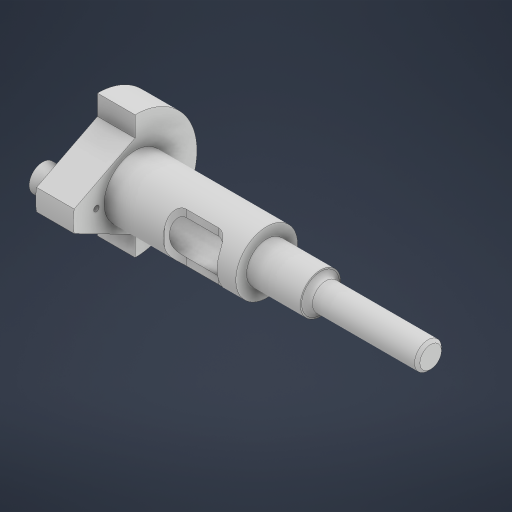
# Autodesk Inventor part: Part4
Saved by Autodesk Inventor 2023 (Build 270158000, 158)
## iProperties
Created: 2023-04-25
Part Number: Part4
Material: Ogólny
Document SubType Name: Modeling
Designer: Adam
Density: 1 g/cm^3
Appearance: Domyślna
Author: Adam
Autodesk Inventor part; units mm, degrees
ref_plane "YZ Plane" through (0, 0, 0) normal (1, 0, 0) x (0, 1, 0)
ref_plane "XZ Plane" through (0, 0, 0) normal (0, 1, 0) x (-1, 0, 0)
ref_plane "XY Plane" through (0, 0, 0) normal (0, 0, 1) x (1, 0, 0)
sketch "Szkic1" plane through (0, 0, 0) normal (0, 0, 1) x (1, 0, 0)
  line L0 (0, 0) -> (14, 0)
  line L1 (14, 0) -> (14, 23)
  line L2 (14, 23) -> (0, 23)
  line L3 (0, 23) -> (0, 0)
  line L4 (14, 0) -> (63, 0)
  line L5 (63, 0) -> (63, 11.5)
  line L6 (63, 11.5) -> (14, 11.5)
  line L7 (14, 11.5) -> (14, 0)
  line L8 (63, 0) -> (83, 0)
  line L9 (83, 0) -> (83, 7.5)
  line L10 (83, 7.5) -> (63, 7.5)
  line L11 (63, 7.5) -> (63, 0)
  line L12 (83, 0) -> (124, 0)
  line L13 (124, 0) -> (124, 5)
  line L14 (124, 5) -> (83, 5)
  line L15 (83, 5) -> (83, 0)
  point P0 (14, 11.5)
  dimension "d0" = 14
  dimension "d1" = 23
  dimension "d2" = 49
  dimension "d3" = 11.5
  dimension "d4" = 20
  dimension "d5" = 7.5
  dimension "d6" = 41
  dimension "d7" = 5
  constraints: 32 end point, 8 parallel, 4 horizontal, 4 perpendicular
  measures "d0" distance of L2.end L1.end
  measures "d1" distance of L1.end L0.end
  measures "d2" distance of L6.end L5.end
  measures "d3" distance of L5.end L4.end
  measures "d4" distance of L10.end L9.end
  measures "d5" distance of L9.end L8.end
  measures "d6" distance of L14.end L13.end
  measures "d7" distance of L13.end L12.end
revolve "Obrót1" add sketch "Szkic1" angle 360 mid plane about axis through (14, 0, 0) along (1, 0, 0)
sketch "Szkic2" plane through (0, 0, 0) normal (-1, 0, 0) x (0, 0, 1)
  circle A0 centre (0, 0) radius 23 projected
  constraints: 1 coincident
hole "Otwór1" at (0, 0, 0) direction (1, 0, 0) diameter 19 depth 57 tip angle 118
chamfer "Faza1" distance 1 angle 45 1 edges at (124, 5, 0) measured on face at (124, 0.8193, 0.3214)
fillet "Zaokrąglenie powierzchni1" radius 2 1 edges at (83, 5, 0)
sketch "Szkic3" plane through (0, 0, 0) normal (1, 0, 0) x (0, 1, 0)
  circle A0 centre (0, 0) radius 23 projected
  line L0 (23, 0) -> (15.5, 0)
  line L1 (15.5, 0) -> (3.9555, 22.6573)
  line L2 (-23, 0) -> (-15.5, 0)
  line L3 (-15.5, 0) -> (-3.9555, 22.6573)
  line L4 (-15.5, 0) -> (9.9289, 0) construction
  dimension "d20" = 7.5
  dimension "d21" = 117
  dimension "d22" = 7.5
  dimension "d23" = 63
  constraints: 10 end point, 4 point on circle, 2 horizontal, 2 point on line, 1 equal length
  measures "d20" distance of L0.start L0.end
  measures "d21" angle of L0 L1
  measures "d22" distance of L2.start L2.end
  measures "d23" angle of L4 L3
extrude "Wyciągnięcie proste1" cut sketch "Szkic3" along normal blind 14 contours L0 L1 A0 | A0 L3 L2
sketch "Szkic4" plane through (0, 0, 0) normal (1, 0, 0) x (0, 1, 0)
  circle A0 centre (0, 14.411) radius 5
  point P0 (0, 0)
  dimension "d26" = 10
  constraints: 1 centre point, 1 coincident
  measures "d26" diameter of A0
extrude "Wyciągnięcie proste2" add sketch "Szkic4" against normal blind 6
sketch "Szkic5" plane through (-6, 0, 14.411) normal (-1, 0, 0) x (0, 0, 1)
  point P0 (-14.411, 0)
  point P1 (0, 0)
hole "Otwór2" at (-6, 0, 14.411) direction (1, 0, 0) diameter 2 end through all
sketch "Szkic6" plane through (0, 0, 0) normal (0, 1, 0) x (-1, 0, 0)
  line L0 (-14, 11.5) -> (-63, 11.5) projected
  line L1 (-40, 7) -> (-52, 7)
  line L2 (-56, 11) -> (-56, 11.5)
  line L3 (-56, 11.5) -> (-36, 11.5)
  line L4 (-36, 11.5) -> (-36, 11)
  line L5 (0, 0) -> (0, 22.6573) projected
  arc A0 (-40, 7) -> (-36, 11) centre (-40, 11) ccw
  arc A1 (-56, 11) -> (-52, 7) centre (-52, 11) ccw
  dimension "d36" = 20
  dimension "d37" = 36
  dimension "d38" = 4.5
  dimension "d39" = 4
  dimension "d40" = 4
  constraints: 8 end point, 4 point on circle, 4 tangent, 2 centre point, 2 parallel, 1 horizontal, 1 perpendicular, 1 point on line
  measures "d36" distance of L2.end L3.end
  measures "d37" distance between parallel lines of L4 L5
  measures "d38" distance between parallel lines of L0 L1
  measures "d39" radius of A0
  measures "d40" radius of A1
extrude "Wyciągnięcie proste3" cut sketch "Szkic6" along normal through all both and the other way through all
